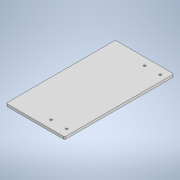
# Autodesk Inventor part: Central Divider
Saved by Autodesk Inventor 2021 (Build 250183000, 183)
## iProperties
Created: 2020-07-14
Part Number: Central Divider
Material: Generic
Document SubType Name: Modeling
Designer: jgray
Density: 1 g/cm^3
Appearance: Default
Author: jgray
Autodesk Inventor part; units mm, degrees
ref_plane "YZ Plane" through (0, 0, 0) normal (1, 0, 0) x (0, 1, 0)
ref_plane "XZ Plane" through (0, 0, 0) normal (0, 1, 0) x (-1, 0, 0)
ref_plane "XY Plane" through (0, 0, 0) normal (0, 0, 1) x (1, 0, 0)
sketch "Sketch1" plane through (0, 0, 0) normal (0, 1, 0) x (-1, 0, 0)
  line L0 (0, 0) -> (111.2, 0)
  line L1 (116.2, 0) -> (116.2, -217)
  line L2 (116.2, -217) -> (0, -217)
  line L3 (0, -217) -> (0, 0)
  line L4 (111.2, 0) -> (111.2, 0)
  line L5 (111.2, 0) -> (116.2, 0)
  dimension "d4" = 5
  dimension "d5" = 111.2
  dimension "d6" = 217
  dimension "d7" = 217
  constraints: 12 end point, 2 parallel, 1 horizontal, 1 perpendicular
  measures "d4" distance of L4.end L1.start
  measures "d5" distance of L0.start L0.end
  measures "d6" distance of L1.start L1.end
  measures "d7" distance of L2.end L0.start
extrude "Extrusion1" add sketch "Sketch1" along normal blind 5
fillet "Fillet1" radius 2 5 edges at (-111.2, 2.5, 0) (0, 2.5, 0) (-116.2, 2.5, 0) (0, 2.5, -217) (-116.2, 2.5, -217)
sketch "Sketch2" plane through (0, 5, 0) normal (0, 1, 0) x (1, 0, 0)
  line L0 (-12, -58.0921) -> (-12, 320.7627) construction
  line L1 (-43, -58.0921) -> (-43, 320.7627) construction
  line L2 (-149.1257, 202) -> (35.6079, 202) construction
  line L3 (-154.8253, 16) -> (27.8967, 16) construction
  line L4 (-114.2, 16) -> (-113.2, 16) construction
  line L5 (0, 2) -> (0, 215) projected
  point P0 (0, 0)
  point P1 (-43, 16)
  point P2 (-12, 16)
  point P3 (-43, 202)
  point P4 (-12, 202)
  dimension "d12" = 186
  dimension "d20" = 12
  dimension "d21" = 31
  constraints: 8 end point, 8 point on line, 2 horizontal, 2 vertical
  measures "d12" distance between parallel lines of L2 L3
  measures "d20" distance between parallel lines of L5 L0
  measures "d21" distance between parallel lines of L0 L1
hole "Hole1" at (-43, 5, -16) at (-12, 5, -16) at (-43, 5, -202) at (-12, 5, -202) direction (0, -1, 0) diameter 4 end through all
body "Solid1"
